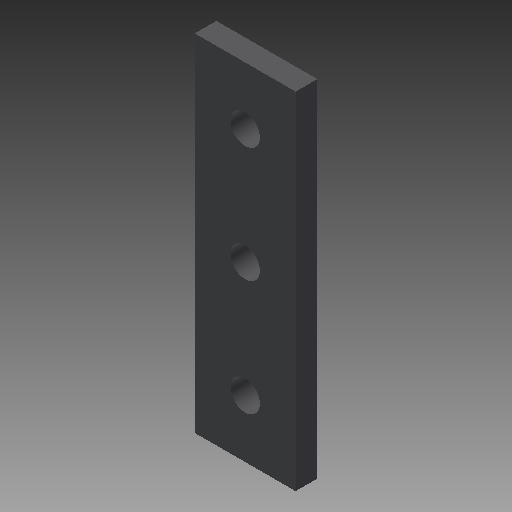
# Autodesk Inventor part: 4118
Saved by Autodesk Inventor 2017 SP1 (Build 210196100, 196)
## iProperties
Category: PARTsolutions
Company: 8020
Created: 2016-04-09
Part Number: 4118
Catalog Web Link: www.cadenas.de
Description: 4118, 4306-Joining Plates - 3 Hole Joining Strip
Vendor: 8020
Document SubType Name: Modeling
Designer: psAdmin
Manufacturer: 8020
Mass: 7.60757 g
Surface Area: 44.2007 cm^2
Volume: 7.60757 cm^3
Density: 1 g/cm^3
Material: Generic
Appearance: PSOLRGB-175-175-175
PSOL_IDENT_0: {$CADENAS_DATA\23d-libs\8020\inch\joining_plates\4118.prj},145 {VTYP=3D},{NB=4118},{LINA=4118},{NN=4
PSOL_IDENT_1: 118, 4306},{DATE=22.08.2012},{GEOMDATE=22.11.2011 11:21:00},{VERSION=},{LINEID=10},{LINESUBID=-1},{W
PSOL_IDENT_2: BVAR=}  {NB=4118},{LINA=4118},{KT=DUMMY},{PN=4118},{A=0.875},{B=3.000},{F=0.257},{W=.045},{A1=0.4375
PSOL_IDENT_3: },{C1=1.500},{C2=0.500},{C3=2.500},{D1=0.188}
NN: 4118, 4306
NT: Joining Plates - 3 Hole Joining Strip
NB: 4118
NBSYN: $PN.
LINA: 4118
PN: 4118
A: 0.875
B: 3.000
W: .045
SUPPLIER: 8020
ARTICLENO: 4118
BOMINFO: 4118
CREATOR: CADENAS GmbH
Title: 4118
Author: Cadenas PARTsolutions
Comments: Joining Plates - 3 Hole Joining Strip
Autodesk Inventor part; units mm, degrees
ref_plane "YZ Plane" through (0, 0, 0) normal (1, 0, 0) x (0, 1, 0)
ref_plane "XZ Plane" through (0, 0, 0) normal (0, 1, 0) x (-1, 0, 0)
ref_plane "XY Plane" through (0, 0, 0) normal (0, 0, 1) x (1, 0, 0)
sketch "Sketch_1" plane through (0, 0, 0) normal (0, 0, 1) x (1, 0, 0)
  line L0 (-11.1125, 76.2) -> (-11.1125, 0)
  line L1 (-11.1125, 0) -> (11.1125, 0)
  line L2 (11.1125, 0) -> (11.1125, 76.2)
  line L3 (11.1125, 76.2) -> (-11.1125, 76.2)
  circle A0 centre (0, 12.7) radius 3.2639
  circle A1 centre (0, 38.1) radius 3.2639
  circle A2 centre (0, 63.5) radius 3.2639
  constraints: 8 end point, 3 centre point
extrude "Extrusion1" add sketch "Sketch_1" along normal blind 4.7752
body "Solid1"
